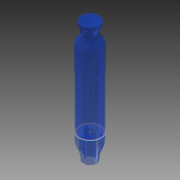
# Autodesk Inventor part: Handle_0
Saved by Autodesk Inventor 2011 SP2 (Build 150309200, 309)
## iProperties
Created: 2012-02-26
Part Number: Handle_0
Document SubType Name: Modeling
Designer: sungwook
Density: 1 g/cm^3
Author: sungwook
Autodesk Inventor part; units mm, degrees
ref_plane "YZ Plane" through (0, 0, 0) normal (1, 0, 0) x (0, 1, 0)
ref_plane "XZ Plane" through (0, 0, 0) normal (0, 1, 0) x (-1, 0, 0)
ref_plane "XY Plane" through (0, 0, 0) normal (0, 0, 1) x (1, 0, 0)
sketch "Sketch2" plane through (0, 0, 0) normal (1, 0, 0) x (0, 1, 0)
  line L0 (0, -35.286548) -> (0, 36.719287)
  line L1 (-12.5, 0) -> (12, 0)
  line L2 (-12.5, 0) -> (-13.516, 0)
  line L3 (-11, 25) -> (0, 25)
  line L4 (11, 25) -> (11, 23.984)
  line L5 (-11, 23.984) -> (-11, 25)
  line L6 (-8.5, 10) -> (8.5, 10)
  line L7 (8.5, 10) -> (8.5, 0)
  line L8 (8.5, 0) -> (-8.5, 0)
  line L9 (-8.5, 0) -> (-8.5, 10)
  line L10 (-12, 5) -> (12, 5)
  line L11 (12, 5) -> (12, 0)
  line L12 (12, 0) -> (-12, 0)
  line L13 (-12, 0) -> (-12, 5)
  line L14 (-7.484, 10) -> (-7.484, 0)
  line L15 (-10.984, 5) -> (-10.984, 0)
  spline S0 degree 4 poles (-11, 23.984) (-11, 20.713142) (-6.85797, 12.864699) (-8.031776, 10.378457) (-11.114983, 5.720869) (-13.616764, 3.542699) (-13.516, 1.361245) (-13.516, 0) knots 0 0 0 0 0 0.40402139 0.58699222 0.72646694 1 1 1 1 1
  spline S1 degree 4 poles (-9.970682, 23.598634) (-9.674097, 19.196604) (-2.8609, 8.377148) (-11.415467, 7.371379) (-12.5, 2.264366) (-12.5, 0) knots 0 0 0 0 0 0.54225417 1 1 1 1 1
  line L16 (-10.208157, 7.245893) -> (-13.791843, 2.754107) construction
  arc A0 (-10.454022, 6.677089) -> (-13.291851, 3.12016) centre (0.50978, -4.980693) ccw construction
  line L17 (-7.766531, 11.715278) -> (-9.233469, 8.284722) construction
  line L18 (0, 23.984) -> (0, 25)
  line L19 (-12.5, 0) -> (-12.5, -25)
  line L20 (-13.516, 0) -> (-13.516, -25)
  arc A1 (-9.484, 23.984) -> (-9.970682, 23.598634) centre (-9.484, 23.484) ccw
  line L21 (-10.161628, 26.432739) -> (-9.779735, 20.764528) construction
  arc A2 (-9.809782, 25.797972) -> (-9.516216, 21.440755) centre (-2.103809, 24.12866) ccw construction
  line L22 (0, 23.984) -> (-9.484, 23.984)
  line L23 (-10.984, 23.984) -> (-11, 23.984)
  line L24 (-13.516, -25) -> (-12.5, -25)
  point P0 (0, 0)
  point P1 (0, 0)
  point P2 (0, 10)
  point P3 (-14.486375, 12.559831)
  point P4 (-9.223277, 8.727179)
  point P5 (-8.085127, 11.403952)
  dimension "d15" = 22
  dimension "d16" = 25
  dimension "d17" = 17
  dimension "d18" = 10
  dimension "d19" = 24
  dimension "d20" = 5
  dimension "d22" = 1.016
  dimension "d23" = 1.016
  dimension "d25" = 1
  dimension "d26" = 25
  dimension "d27" = 1.016
  dimension "d28" = 12.5
  constraints: 48 end point, 11 parallel, 9 midpoint, 7 point on line, 5 horizontal, 5 perpendicular, 4 coincident, 4 point on circle, 3 centre point, 3 vertical, 2 tangent, 2 vertical alignment, 18 other
  measures "d15" distance of L4.start L3.start
  measures "d16" distance between parallel lines of L1 L3
  measures "d17" distance between parallel lines of L7 L9
  measures "d18" distance between parallel lines of L8 L6
  measures "d19" distance between parallel lines of L11 L13
  measures "d20" distance between parallel lines of L12 L10
  measures "d22" distance between parallel lines of L14 L9
  measures "d23" distance between parallel lines of L15 L13
  measures "d25" diameter of A1
  measures "d26" distance of L20.end L2.end
  measures "d27" distance of L1.start L2.end
  measures "d28" distance of point (0, 0) L1.start
revolve "Revolution1" add sketch "Sketch2" angle 360 about axis through (0, 0, -10) along (0, 0, 1) contours L22 A1 S1 L6 S0 L5 L3 L0 | S1 L9 L6 | L9 S1 L10 S0 | L10 S1 L13 | L13 S1 L2 S0
revolve "Revolution2" add sketch "Sketch2" angle 360 about axis through (0, 0, -10) along (0, 0, 1) contours L2 L19 L24 L20
sketch "Sketch4" plane through (0, 0, 0) normal (1, 0, 0) x (0, 1, 0)
  line L0 (-13.516, -25) -> (-13.516, 0)
  line L1 (-12.5, 0) -> (-12.5, -25)
  line L2 (13.516, -25) -> (-13.516, -25)
  line L3 (0, -36.032013) -> (0, 6.005335)
  line L4 (-12, -25) -> (12, -25)
  line L5 (12, -25) -> (12, -29.976908)
  line L6 (12, -29.976908) -> (-12, -29.976908)
  line L7 (-12, -29.976908) -> (-12, -25)
  line L8 (-12, -29.976908) -> (-13.016, -29.976908)
  line L9 (-12, -25) -> (-12, -29.976908)
  spline S0 degree 4 poles (-12, -29.976908) (-12, -29.350097) (-12, -28.096475) (-12.5, -26.880433) (-12.5, -25.626811) (-12.5, -25) knots 0 0 0 0 0 0.5 1 1 1 1 1
  spline S1 degree 4 poles (-13.016, -29.976908) (-13.016, -29.350097) (-13.016, -28.096475) (-13.516, -26.880433) (-13.516, -25.626811) (-13.516, -25) knots 0 0 0 0 0 0.5 1 1 1 1 1
  point P0 (0, 0)
  point P1 (0, -25)
  point P2 (0, -25)
  point P3 (-13.016, -25)
  dimension "d34" = 24
  dimension "d37" = 1.016
  constraints: 12 end point, 3 vertical, 2 horizontal, 2 midpoint, 2 parallel, 2 point on line, 1 coincident, 1 perpendicular, 4 other
  measures "d34" distance between parallel lines of L5 L7
  measures "d37" distance of L6.end L8.end
sketch "Sketch4 outline for Revolution4" plane through (0, 0, 0) normal (1, 0, 0) x (0, 1, 0)
  spline S0 degree 4 poles (-13.016, -29.976908) (-13.016, -29.350097) (-13.016, -28.096475) (-13.516, -26.880433) (-13.516, -25.626811) (-13.516, -25) knots 0 0 0 0 0 0.5 1 1 1 1 1
  line L0 (-12.5, -25) -> (-13.516, -25)
  spline S1 degree 4 poles (-12, -29.976908) (-12, -29.350097) (-12, -28.096475) (-12.5, -26.880433) (-12.5, -25.626811) (-12.5, -25) knots 0 0 0 0 0 0.5 1 1 1 1 1
  line L1 (-13.016, -29.976908) -> (-12, -29.976908)
revolve "Revolution4" add sketch "Sketch4 outline for Revolution4" angle 360 about axis through (0, 0, -10) along (0, 0, 1)
sketch "Sketch5" plane through (0, 0, 0) normal (1, 0, 0) x (0, 1, 0)
  line L0 (13.016, -29.976908) -> (-13.016, -29.976908)
  line L1 (12, -29.976908) -> (-12, -29.976908)
  line L2 (0, -107.97229) -> (0, 17.995382)
  line L3 (-12, -29.976908) -> (12, -29.976908)
  line L4 (12, -29.976908) -> (12, -89.976908)
  line L5 (12, -89.976908) -> (-12, -89.976908)
  line L6 (-12, -89.976908) -> (-12, -29.976908)
  line L7 (-12, -29.976908) -> (-13.016, -29.976908)
  line L8 (-12, -89.976908) -> (-13.016, -89.976908)
  line L9 (-13.016, -89.976908) -> (-13.016, -29.976908)
  point P0 (0, 0)
  dimension "d39" = 24
  dimension "d40" = 1.016
  dimension "d41" = 60
  constraints: 14 end point, 3 parallel, 2 perpendicular, 1 horizontal
  measures "d39" distance between parallel lines of L4 L6
  measures "d40" distance of L5.end L8.end
  measures "d41" distance between parallel lines of L5 L0
revolve "Revolution5" add sketch "Sketch5" angle 360 about axis through (0, 0, -10) along (0, 0, 1) contours L6 L8 L9 L0
sketch "Sketch7" plane through (0, 0, -89.976908) normal (0, 0, -1) x (-1, 0, 0)
  circle A0 centre (0, 0) radius 13.016 projected
  circle A1 centre (0, 0) radius 12 projected
  circle A2 centre (0, 0) radius 13.016
  constraints: 1 centre point, 1 coincident, 1 concentric
ref_plane "Work Plane5" through (0, 0, -89.976908) normal (0, 0, 1) x (1, 0, 0)
extrude "Extrusion1" add sketch "Sketch7" along normal blind 4 contours A0 | A1
sketch "Sketch8" plane through (0, 0, -93.976908) normal (0, 0, -1) x (-1, 0, 0)
  circle A0 centre (0, 0) radius 13.016
  line L0 (7.582299, 2.074) -> (6.427599, 4.074)
  line L1 (6.427599, 4.074) -> (7.582299, 6.074)
  line L2 (7.582299, 6.074) -> (9.891701, 6.074)
  line L3 (9.891701, 6.074) -> (11.046401, 4.074)
  line L4 (11.046401, 4.074) -> (9.891701, 2.074)
  line L5 (9.891701, 2.074) -> (7.582299, 2.074)
  line L6 (0, -19.012167) -> (0, 19.012167)
  line L7 (-9.503701, 6.82) -> (-7.194299, 6.82)
  line L8 (-7.194299, 6.82) -> (-6.039599, 4.82)
  line L9 (-6.039599, 4.82) -> (-7.194299, 2.82)
  line L10 (-7.194299, 2.82) -> (-9.503701, 2.82)
  line L11 (-9.503701, 2.82) -> (-10.658401, 4.82)
  line L12 (-10.658401, 4.82) -> (-9.503701, 6.82)
  line L13 (1.154701, -7.494) -> (2.309401, -9.494)
  line L14 (2.309401, -9.494) -> (1.154701, -11.494)
  line L15 (1.154701, -11.494) -> (-1.154701, -11.494)
  line L16 (-1.154701, -11.494) -> (-2.309401, -9.494)
  line L17 (-2.309401, -9.494) -> (-1.154701, -7.494)
  line L18 (-1.154701, -7.494) -> (1.154701, -7.494)
  point P0 (8.737, 4.074)
  point P1 (-8.349, 4.82)
  point P2 (0, -9.494)
  point P3 (8.737, 4.074)
  dimension "d45" = 4.074
  dimension "d46" = 8.737
  dimension "d47" = 4.82
  dimension "d48" = 8.349
  dimension "d49" = 9.494
  dimension "d51" = 4
  dimension "d52" = 4
  dimension "d53" = 4
  constraints: 36 end point, 1 coincident, 1 other
  measures "d45" vertical distance of point (8.737, 4.074) A0.centre
  measures "d46" horizontal distance of point (8.737, 4.074) A0.centre
  measures "d47" vertical distance of point (-8.349, 4.82) A0.centre
  measures "d48" horizontal distance of A0.centre point (-8.349, 4.82)
  measures "d49" distance of point (0, -9.494) A0.centre
  measures "d51" distance between parallel lines of L0 L3
  measures "d52" distance between parallel lines of L7 L10
  measures "d53" distance between parallel lines of L13 L16
hole "Hole1" at (-8.737, 4.074, -93.976908) at (8.349, 4.82, -93.976908) at (0, -9.494, -93.976908) at (-8.737, 4.074, -93.976908) direction (0, 0, 1) diameter 1.778 depth 4 clearance for "Flat Head Machine Screw (82)" size "#0" standard "Ansi Unified Screw Threads"
sketch "Sketch9" plane through (0, 0, 0) normal (1, 0, 0) x (0, 1, 0)
  line L0 (-13.016, -93.976908) -> (-13.016, -29.976908)
  line L1 (13.016, -93.976908) -> (-13.016, -93.976908)
  line L2 (0, -143.07229) -> (0, 23.845382)
  line L3 (-8, -93.976908) -> (0, -93.976908)
  line L4 (0, -93.976908) -> (0, -118.976908)
  line L5 (0, -118.976908) -> (-8, -118.976908)
  spline S0 degree 4 poles (-13.016, -93.976908) (-13.016, -97.195328) (-13.016, -103.632168) (-8, -109.321648) (-8, -115.758488) (-8, -118.976908) knots 0 0 0 0 0 0.5 1 1 1 1 1
  line L6 (-13.016, -93.976908) -> (-8, -93.976908)
  point P0 (0, 0)
  point P1 (-4, -93.976908)
  dimension "d68" = 25
  constraints: 8 end point, 2 midpoint, 1 coincident, 1 horizontal, 1 horizontal alignment, 1 parallel, 1 perpendicular, 1 vertical, 2 other
  measures "d68" distance between parallel lines of L5 L3
revolve "Revolution6" add sketch "Sketch9" angle 360 about axis through (0, 0, -10) along (0, 0, 1)
ref_plane "Work Plane6" through (0, 0, -92.476908) normal (0, 0, 1) x (1, 0, 0)
sketch "Sketch11" plane through (0, 0, -92.476908) normal (0, 0, 1) x (1, 0, 0)
  circle A0 centre (-8.737, 4.074) radius 0.889
  circle A1 centre (8.349, 4.82) radius 0.889
  circle A2 centre (0, -9.494) radius 0.889
  line L0 (-9.891701, 2.074) -> (-7.582299, 2.074)
  line L1 (-11.046401, 4.074) -> (-9.891701, 2.074)
  line L2 (-7.582299, 2.074) -> (-6.427599, 4.074)
  line L3 (-9.891701, 6.074) -> (-11.046401, 4.074)
  line L4 (-7.582299, 6.074) -> (-9.891701, 6.074)
  line L5 (-6.427599, 4.074) -> (-7.582299, 6.074)
  line L6 (1.154701, -7.494) -> (-1.154701, -7.494)
  line L7 (2.309401, -9.494) -> (1.154701, -7.494)
  line L8 (1.154701, -11.494) -> (2.309401, -9.494)
  line L9 (-1.154701, -11.494) -> (1.154701, -11.494)
  line L10 (-2.309401, -9.494) -> (-1.154701, -11.494)
  line L11 (-1.154701, -7.494) -> (-2.309401, -9.494)
  line L12 (7.194299, 6.82) -> (6.039599, 4.82)
  line L13 (9.503701, 6.82) -> (7.194299, 6.82)
  line L14 (10.658401, 4.82) -> (9.503701, 6.82)
  line L15 (9.503701, 2.82) -> (10.658401, 4.82)
  line L16 (7.194299, 2.82) -> (9.503701, 2.82)
  line L17 (6.039599, 4.82) -> (7.194299, 2.82)
  point P0 (0, 0)
extrude "Extrusion3" cut sketch "Sketch11" against normal through all contours A0 | A1 | A2 | L1 L3 L4 L5 L2 L0 | L7 L8 L9 L10 L11 L6 | L13 L14 L15 L16 L17 L12
ref_plane "Work Plane7" through (0, 0, -89.976908) normal (0, 0, 1) x (1, 0, 0)
hole "Hole2" at (0, 0, -118.976908) direction (0, 0, 1) diameter 10 depth 29
equation "\"d22\" = d24"
equation "\"d23\" = d24"
equation "\"d27\" = t"
equation "\"d37\" = t"
equation "\"d40\" = t"
equation "\"t\" = 1.016"
equation "\"d14\" = d24"
equation "\"d24\" = 1.016"
body "Solid1"
